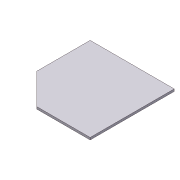
# Autodesk Inventor part: camera_hole_tape
Saved by Autodesk Inventor 2014 SP1 (Build 180222100, 222)
## iProperties
Created: 2013-06-08
Material: Aluminum-6061
Document SubType Name: Modeling
Designer: Robert Davis
Mass: 0.491733 g
Surface Area: 7.63905 cm^2
Volume: 0.181451 cm^3
Density: 2.71 g/cm^3
Description: 1ST SURF METAL TAPE
Appearance: Aluminum - Flat
Author: Robert Davis
Autodesk Inventor part; units mm, degrees
ref_plane "YZ Plane" through (0, 0, 0) normal (1, 0, 0) x (0, 1, 0)
sketch "Sketch1" plane through (0, 0, 0) normal (0, 0, 1) x (1, 0, 0)
  line L0 (-9.525, 9.525) -> (9.525, 9.525)
  line L1 (9.525, 9.525) -> (9.525, -9.525)
  line L2 (9.525, -9.525) -> (-9.525, -9.525)
  line L3 (-9.525, -9.525) -> (-9.525, 9.525)
  line L4 (0, 4.9747) -> (0, 0)
  line L5 (0, 0) -> (3.911, 0)
  dimension "d0" = 19.05
  dimension "d1" = 19.05
  constraints: 12 end point, 3 horizontal, 3 vertical, 1 coincident, 2 other
  measures "d0" distance of L0.start L0.end
  measures "d1" distance of L0.end L1.end
extrude "Extrusion1" add sketch "Sketch1" along normal blind 0.5
ref_plane "Work Plane1" through (-9.525, -9.525, 0) normal (-0.7071, 0.7071, 0) x (0, 0, 1)
ref_plane "Work Plane2" through (9.525, -9.525, 0) normal (-0.7071, -0.7071, 0) x (0, 0, 1)
chamfer "Chamfer1" distance 7 angle 45 1 edges at (-9.525, -9.525, 0.25)
body "Solid1"
